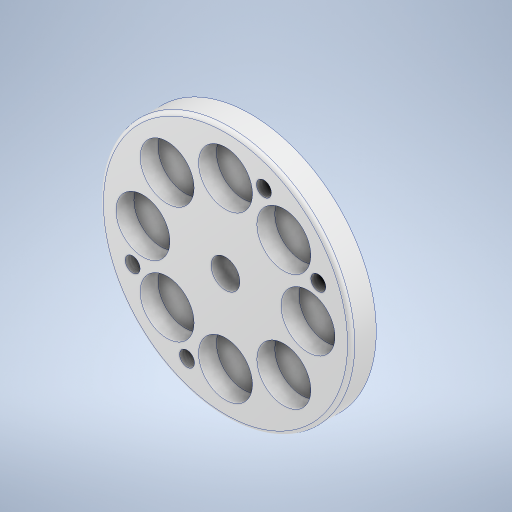
# Autodesk Inventor part: P003
Saved by Autodesk Inventor 2023 (Build 270158000, 158)
## iProperties
Created: 2022-08-22
Part Number: P003
Material: Aluminum 6061
Document SubType Name: Modeling
Designer: D.C. Eksteen
Density: 2.7 g/cm^3
Appearance: Aluminum - Flat
Mass: 62.3992 g
Surface Area: 114.065 cm^2
Volume: 23.1108 cm^3
Author: D.C. Eksteen
Title: POSITIONING MAGNET DISC
Autodesk Inventor part; units mm, degrees
sketch "Sketch1" plane through (0, 0, 0) normal (0, 0, 1) x (1, 0, 0)
  circle A0 centre (0, 0) radius 35
  dimension "d0" = 70
  constraints: 1 centre point, 1 coincident
  measures "d0" diameter of A0
extrude "Extrusion1" add sketch "Sketch1" along normal blind 7
sketch "Sketch2" plane through (0, 0, 7) normal (0, 0, 1) x (1, 0, 0)
  circle A0 centre (0, 0) radius 35 projected
  circle A1 centre (0, 0) radius 23 construction
  line L0 (0, 0) -> (0, 23) construction
  point P0 (-16.2635, 16.2635)
  point P1 (-23, 0)
  point P2 (-16.2635, -16.2635)
  point P3 (0, -23)
  point P4 (16.2635, -16.2635)
  point P5 (23, 0)
  point P6 (16.2635, 16.2635)
  dimension "d3" = 46
  dimension "d6" = 360
  constraints: 2 end point, 1 coincident, 1 vertical, 1 vertical alignment, 11 other
hole "Hole1" at (0, 23, 7) at (-16.2635, 16.2635, 7) at (-23, 0, 7) at (-16.2635, -16.2635, 7) at (0, -23, 7) at (16.2635, -16.2635, 7) at (23, 0, 7) at (16.2635, 16.2635, 7) direction (0, 0, -1) diameter 15 depth 5
fillet "Fillet2" radius 1 1 edges at (-35, 0, 7)
sketch "Sketch12" plane through (0, 0, 0) normal (0, 0, -1) x (-1, 0, 0)
  circle A0 centre (0, 0) radius 35 projected
  circle A1 centre (0, 0) radius 11
  dimension "d62" = 22
  constraints: 1 centre point, 1 coincident
  measures "d62" diameter of A1
extrude "Extrusion4" add sketch "Sketch12" along normal blind 10 contours A1
sketch "Sketch13" plane through (0, 0, -10) normal (0, 0, -1) x (-1, 0, 0)
  point P0 (0, 0)
  point P1 (0, 0)
  constraints: 1 coincident
hole "Hole6" at (0, 0, -10) direction (0, 0, 1) diameter 8 end through all
sketch "Sketch14" plane through (0, 0, 7) normal (0, 0, 1) x (1, 0, 0)
  circle A0 centre (0, 0) radius 28 construction
  circle A1 centre (0, 0) radius 4 projected
  circle A2 centre (16.2635, 16.2635) radius 7.5 projected
  circle A3 centre (16.2635, -16.2635) radius 7.5 projected
  circle A4 centre (-16.2635, -16.2635) radius 7.5 projected
  circle A5 centre (-16.2635, 16.2635) radius 7.5 projected
  circle A6 centre (0, 23) radius 7.5 projected
  circle A7 centre (-23, 0) radius 7.5 projected
  circle A8 centre (0, -23) radius 7.5 projected
  circle A9 centre (23, 0) radius 7.5 projected
  circle A10 centre (0, 0) radius 34 projected
  circle A11 centre (0, 0) radius 4 projected
  line L0 (0, 0) -> (16.2635, 16.2635)
  line L1 (0, 0) -> (10.7151, 25.8686)
  line L2 (25.8686, 10.7151) -> (0, 0)
  line L3 (16.2635, -16.2635) -> (-16.2635, 16.2635)
  point P0 (-25.8686, -10.7151)
  point P1 (-10.7151, -25.8686)
  dimension "d72" = 56
  dimension "d73" = 22.5
  dimension "d74" = 22.5
  constraints: 8 end point, 3 coincident, 2 point on circle, 2 symmetric about line, 1 centre point
  measures "d72" diameter of A0
  measures "d73" angle of L0 L2
  measures "d74" angle of L1 L0
hole "Hole7" at (25.8686, 10.7151, 7) at (10.7151, 25.8686, 7) at (-10.7151, -25.8686, 7) at (-25.8686, -10.7151, 7) direction (0, 0, -1) diameter 4.134 end through all thread size "M5x0.8" class "6H" standard "ANSI Metric M Profile"
ref_plane "Work Plane1" through (0, -11, 0) normal (0, 1, 0) x (-1, 0, 0)
sketch "Sketch15" plane through (0, -11, 0) normal (0, 1, 0) x (-1, 0, 0)
  line L0 (-11, -10) -> (11, -10) projected
  line L1 (11, 0) -> (-11, 0) projected
  line L2 (-11, 0) -> (-11, -10) projected
  line L3 (11, 0) -> (-11, 0)
  line L4 (-11, 0) -> (-11, -3)
  line L5 (-11, -3) -> (11, -3)
  line L6 (11, -3) -> (11, 0)
  point P0 (0, 0)
  point P1 (0, -5)
  dimension "d82" = 3
  dimension "d83" = 11
  dimension "d84" = 5
  constraints: 8 end point, 2 parallel, 1 horizontal, 1 perpendicular, 1 point on line
  measures "d82" distance of L4.end L3.end
  measures "d83" distance from line of L2 point (0, -5)
  measures "d84" distance from line of L0 point (0, -5)
hole "Hole8" at (0, -11, -5) direction (0, 1, 0) diameter 3.242 depth 11.05 tip angle 118 thread size "M4x0.7" class "6H" standard "ANSI Metric M Profile"
sketch "Sketch16" plane through (0, 0, -10) normal (0, 0, -1) x (-1, 0, 0)
  circle A0 centre (0, 0) radius 4 projected
  circle A1 centre (0, 0) radius 11 projected
  line L0 (0, 0) -> (0, -11)
  circle A2 centre (0, 0) radius 11 projected
  line L1 (0, 0) -> (-9.5263, 5.5)
  line L2 (0, 0) -> (9.5263, 5.5)
  dimension "d92" = 120
  dimension "d93" = 120
  constraints: 6 end point, 2 point on circle, 1 vertical, 1 vertical alignment, 1 other
  measures "d92" angle of L1 L0
  measures "d93" angle of L0 L2
ref_plane "Work Plane2" through (9.5263, 5.5, -10) normal (0.866, 0.5, 0) x (-0.5, 0.866, 0)
ref_plane "Work Plane3" through (-9.5263, 5.5, -10) normal (-0.866, 0.5, 0) x (-0.5, -0.866, 0)
sketch "Sketch17" plane through (9.5263, 5.5, -10) normal (0.866, 0.5, 0) x (-0.5, 0.866, 0)
  line L0 (35, 10) -> (-35, 10) projected
  line L1 (35, 16) -> (-35, 16) projected
  line L2 (-11, 0) -> (11, 0) projected
  line L3 (11, 10) -> (11, 0) projected
  line L4 (-11, 10) -> (-11, 0) projected
  point P0 (0, 10)
  point P1 (0, 5)
  dimension "d94" = 11
  dimension "d95" = 5
  measures "d94" distance from line of L4 point (0, 5)
  measures "d95" distance from line of L0 point (0, 5)
hole "Hole9" at (9.5263, 5.5, -5) direction (-0.866, -0.5, 0) diameter 3.242 depth 11.05 tip angle 118 thread size "M4x0.7" class "6H" standard "ANSI Metric M Profile"
sketch "Sketch18" plane through (-9.5263, 5.5, -10) normal (-0.866, 0.5, 0) x (-0.5, -0.866, 0)
  line L0 (11, 10) -> (11, 0) projected
  line L1 (35, 10) -> (-35, 10) projected
  line L2 (-11, 0) -> (11, 0) projected
  line L3 (-11, 10) -> (-11, 0) projected
  point P0 (0, 10)
  point P1 (0, 5)
  dimension "d103" = 5
  dimension "d104" = 11
  measures "d103" distance from line of L1 point (0, 5)
  measures "d104" distance from line of L3 point (0, 5)
hole "Hole10" at (-9.5263, 5.5, -5) direction (0.866, -0.5, 0) diameter 3.242 depth 11.05 tip angle 118 thread size "M4x0.7" class "6H" standard "ANSI Metric M Profile"
body "Solid1"
